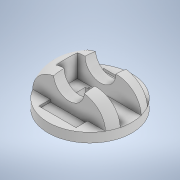
# Autodesk Inventor part: Baserotate
Saved by Autodesk Inventor 2022 (Build 260153000, 153)
## iProperties
Created: 2022-01-07
Part Number: Baserotate
Material: Generic
Document SubType Name: Modeling
Designer: nguye
Density: 1 g/cm^3
Appearance: Default
Author: nguye
Autodesk Inventor part; units mm, degrees
ref_plane "YZ Plane" through (0, 0, 0) normal (1, 0, 0) x (0, 1, 0)
ref_plane "XZ Plane" through (0, 0, 0) normal (0, 1, 0) x (-1, 0, 0)
ref_plane "XY Plane" through (0, 0, 0) normal (0, 0, 1) x (1, 0, 0)
sketch "Sketch1" plane through (0, 0, 0) normal (0, 1, 0) x (-1, 0, 0)
  circle A0 centre (0, 0) radius 90
  dimension "d0" = 180
  constraints: 1 centre point, 1 coincident
  measures "d0" diameter of A0
extrude "Extrusion1" add sketch "Sketch1" along normal blind 100
sketch "Sketch2" plane through (0, 100, 0) normal (0, 1, 0) x (1, 0, 0)
  circle A0 centre (0, 0) radius 90 projected
  line L0 (0, -90) -> (-90, -90)
  line L1 (-90, -90) -> (-90, -45)
  line L2 (-90, -45) -> (0, -45)
  line L3 (0, 90) -> (-90, 90)
  line L4 (-90, 90) -> (-90, 45)
  line L5 (-90, 45) -> (0, 45)
  line L6 (0, -90) -> (90, -90)
  line L7 (90, -90) -> (90, -45)
  line L8 (90, -45) -> (0, -45)
  line L9 (0, 90) -> (90, 90)
  line L10 (90, 90) -> (90, 45)
  line L11 (90, 45) -> (0, 45)
  point P0 (77.9423, -45)
  point P1 (-77.9423, -45)
  point P2 (77.9423, 45)
  point P3 (-77.9423, 45)
  dimension "d3" = 45
  dimension "d4" = 45
  dimension "d5" = 90
  dimension "d6" = 90
  constraints: 24 end point, 4 horizontal, 4 parallel, 4 perpendicular, 2 point on circle, 1 point on line
  measures "d3" distance of L0.end L1.end
  measures "d4" distance of L4.end L3.end
  measures "d5" distance of L8.end L7.end
  measures "d6" distance of L10.end L11.end
extrude "Extrusion2" cut sketch "Sketch2" against normal blind 60 contours L11 L5 A0 | A0 L2 L8
sketch "Sketch3" plane through (77.9423, 100, -45) normal (0, 0, -1) x (-1, 0, 0)
  line L0 (0, 0) -> (-12.0577, 0) projected
  line L1 (167.9423, -100) -> (167.9423, 0) projected
  line L2 (-12.0577, 0) -> (167.9423, 0)
  line L3 (167.9423, 0) -> (167.9423, -30)
  line L4 (167.9423, -30) -> (-12.0577, -30)
  line L5 (-12.0577, -30) -> (-12.0577, 0)
  point P0 (77.9423, -100)
  dimension "d9" = 30
  constraints: 8 end point, 2 parallel, 1 horizontal, 1 perpendicular, 1 point on line
  measures "d9" distance of L2.end L3.end
extrude "Extrusion3" cut sketch "Sketch3" against normal blind 108.75
sketch "Sketch4" plane through (-77.9423, 70, -45) normal (0, 1, 0) x (1, 0, 0)
  circle A0 centre (77.9423, -45) radius 90 projected
  line L0 (27.9423, -67.5) -> (193.7898, -67.5)
  line L1 (193.7898, -67.5) -> (193.7898, -22.5)
  line L2 (193.7898, -22.5) -> (27.9423, -22.5)
  line L3 (27.9423, -22.5) -> (27.9423, -67.5)
  point P0 (165.0844, -67.5)
  point P1 (165.0844, -22.5)
  constraints: 8 end point, 2 parallel, 1 horizontal, 1 perpendicular
extrude "Extrusion4" cut sketch "Sketch4" against normal blind 50 contours A0 L0 L3 L2 picked at (74.609, -45)
sketch "Sketch5" plane through (0, 40, 0) normal (0, 1, 0) x (1, 0, 0)
  line L0 (-77.9423, 45) -> (77.9423, 45) projected
  line L1 (0, 45) -> (-77.9423, 45)
  line L2 (-77.9423, 45) -> (77.9423, 45)
  line L3 (-77.9423, -45) -> (77.9423, -45) projected
  line L4 (0, -45) -> (-77.9423, -45)
  circle A0 centre (0, 0) radius 90 projected
  line L5 (-77.9423, -45) -> (77.9423, -45)
  arc A1 (-77.9423, -45) -> (77.9423, -45) centre (0, 0) ccw
  arc A2 (77.9423, 45) -> (-77.9423, 45) centre (0, 0) ccw
  constraints: 8 end point, 5 point on circle, 2 centre point, 2 collinear, 2 midpoint, 1 coincident, 1 horizontal, 1 point on line
extrude "Extrusion5" cut sketch "Sketch5" against normal blind 20 contours A0 L0 | L3 A0
fillet "Fillet1" radius 50 2 edges at (83.3053, 70, -34.0621) (-86.9333, 70, -23.2937)
sketch "Sketch6" plane through (-77.9423, 20, -45) normal (0, 1, 0) x (1, 0, 0)
  line L0 (62.9423, -30) -> (77.9423, -30)
  line L1 (92.9423, -30) -> (77.9423, -30)
  line L2 (62.9423, -60) -> (77.9423, -60)
  line L3 (92.9423, -60) -> (77.9423, -60)
  line L4 (62.9423, -60) -> (52.9423, -60)
  line L5 (52.9423, -60) -> (52.9423, -30)
  line L6 (52.9423, -30) -> (62.9423, -30)
  line L7 (92.9423, -30) -> (102.9423, -30)
  line L8 (102.9423, -30) -> (102.9423, -60)
  line L9 (102.9423, -60) -> (92.9423, -60)
  point P0 (77.9423, -45)
  dimension "d21" = 15
  dimension "d23" = 10
  dimension "d24" = 10
  constraints: 20 end point, 2 horizontal, 2 parallel, 2 perpendicular, 1 point on line
  measures "d21" distance of L0.start L0.end
  measures "d23" distance of L5.end L6.end
  measures "d24" distance of L8.end L9.end
extrude "Extrusion6" cut sketch "Sketch6" against normal blind 20
sketch "Sketch7" plane through (77.9423, 20, -45) normal (0, 0, -1) x (-1, 0, 0)
  line L0 (111.0141, 50) -> (44.8704, 50) projected
  circle A0 centre (77.9423, 50) radius 33.0719
  point P0 (77.9423, -20)
  constraints: 1 midpoint, 3 other
extrude "Extrusion7" cut sketch "Sketch7" against normal blind 137.75 contours A0 L0 picked at (67.2386, 47.3618)
sketch "Sketch10" plane through (-77.9423, 20, -45) normal (0, 1, 0) x (1, 0, 0)
  circle A0 centre (57.9423, -62.5) radius 1.5
  line L0 (102.9423, -30) -> (102.9423, -60) projected
  circle A1 centre (97.9423, -62.5) radius 1.5
  circle A2 centre (57.9423, -27.5) radius 1.5
  circle A3 centre (97.9423, -27.5) radius 1.5
  point P0 (77.9423, -45)
  point P1 (52.9423, -60)
  point P2 (52.9423, -30)
  dimension "d34" = 3
  dimension "d37" = 3
  dimension "d40" = 3
  dimension "d43" = 3
  constraints: 4 centre point
  measures "d34" diameter of A0
  measures "d37" diameter of A1
  measures "d40" diameter of A2
  measures "d43" diameter of A3
extrude "Extrusion8" cut sketch "Sketch10" against normal blind 5
sketch "Sketch11" plane through (0, 20, 0) normal (0, 1, 0) x (1, 0, 0)
  line L0 (77.9423, 45) -> (-77.9423, 45) projected
  line L1 (0, 45) -> (-40, 45)
  line L2 (-40, 45) -> (-40, 70)
  line L3 (-40, 70) -> (40, 70)
  line L4 (40, 70) -> (40, 45)
  line L5 (0, 45) -> (40, 45)
  line L6 (-77.9423, -45) -> (77.9423, -45) projected
  line L7 (0, -45) -> (-40, -45)
  line L8 (-40, -45) -> (40, -45)
  line L9 (40, -45) -> (40, -70)
  line L10 (40, -70) -> (-40, -70)
  line L11 (-40, -70) -> (-40, -45)
  point P0 (0, 0)
  dimension "d46" = 40
  dimension "d47" = 25
  dimension "d48" = 80
  dimension "d49" = 80
  dimension "d50" = 25
  constraints: 20 end point, 4 perpendicular, 3 point on line, 2 midpoint, 2 parallel, 1 horizontal, 1 vertical
  measures "d46" distance of L1.start L1.end
  measures "d47" distance of L1.end L2.end
  measures "d48" distance of L2.end L3.end
  measures "d49" distance of L9.end L10.end
  measures "d50" distance of L8.end L9.end
extrude "Extrusion9" cut sketch "Sketch11" against normal blind 5
body "Solid1"
